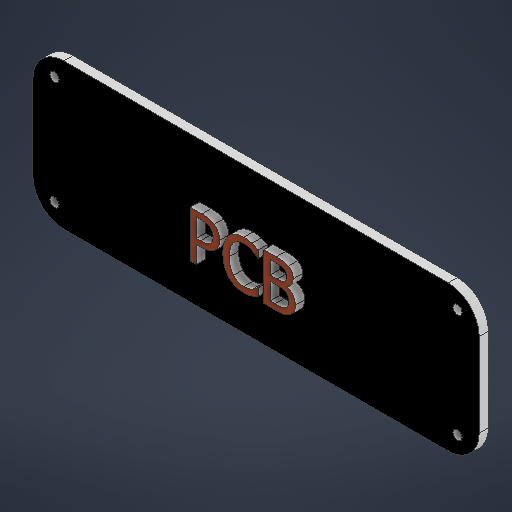
# Autodesk Inventor part: PCB
Saved by Autodesk Inventor 2025 (Build 290162000, 162)
## iProperties
Created: 2024-05-23
Part Number: PCB
Material: Generic
Document SubType Name: Modeling
Designer: techn
Density: 1 g/cm^3
Appearance: Default
Author: techn
Autodesk Inventor part; units mm, degrees
ref_plane "YZ Plane" through (0, 0, 0) normal (1, 0, 0) x (0, 1, 0)
ref_plane "XZ Plane" through (0, 0, 0) normal (0, 1, 0) x (-1, 0, 0)
ref_plane "XY Plane" through (0, 0, 0) normal (0, 0, 1) x (1, 0, 0)
sketch "Sketch1" plane through (0, 0, 0) normal (0, 0, 1) x (1, 0, 0)
  circle A0 centre (0, 0) radius 1.5
  circle A1 centre (0, 0) radius 3
  circle A2 centre (0, 35) radius 1.5
  circle A3 centre (0, 35) radius 3
  circle A4 centre (130, 35) radius 1.5
  circle A5 centre (130, 35) radius 3
  circle A6 centre (130, 0) radius 1.5
  circle A7 centre (130, 0) radius 3
  line L0 (3, 41) -> (127, 41)
  line L1 (137, 31) -> (137, 4)
  line L2 (127, -6) -> (3, -6)
  line L3 (-7, 4) -> (-7, 31)
  arc A8 (3, 41) -> (-7, 31) centre (3, 31) ccw
  arc A9 (-7, 4) -> (3, -6) centre (3, 4) ccw
  arc A10 (127, -6) -> (137, 4) centre (127, 4) ccw
  arc A11 (137, 31) -> (127, 41) centre (127, 31) ccw
  dimension "d0" = 3
  dimension "d1" = 1.5
  dimension "d2" = 3
  dimension "d3" = 1.5
  dimension "d4" = 3
  dimension "d5" = 1.5
  dimension "d6" = 3
  dimension "d7" = 1.5
  dimension "d8" = 130
  dimension "d9" = 35
  dimension "d10" = 7
  dimension "d11" = 6
  dimension "d12" = 6
  dimension "d13" = 7
  dimension "d14" = 10
  constraints: 12 centre point, 8 end point, 8 point on circle, 8 tangent, 3 equal radius, 2 horizontal alignment, 2 parallel, 2 vertical alignment, 1 coincident, 1 horizontal, 1 perpendicular
  measures "d0" diameter of A0
  measures "d1" radial gap between concentric circles of A0 A1
  measures "d2" diameter of A2
  measures "d3" radial gap between concentric circles of A2 A3
  measures "d4" diameter of A4
  measures "d5" radial gap between concentric circles of A4 A5
  measures "d6" diameter of A6
  measures "d7" radial gap between concentric circles of A6 A7
  measures "d8" distance of A6.centre A0.centre
  measures "d9" distance of A0.centre A2.centre
  measures "d10" distance from line of L3 A2.centre
  measures "d11" distance from line of L0 A2.centre
  measures "d12" distance from line of L2 A0.centre
  measures "d13" distance from line of L1 A6.centre
  measures "d14" radius of A8
extrude "Extrusion1" add sketch "Sketch1" along normal blind 3 contours A1 | A3 | A5 | A7 | L0 A11 L1 A10 L2 A9 L3 A8
sketch "Sketch2" plane through (0, 0, 3) normal (0, 0, 1) x (1, 0, 0)
  line L0 (45.2495, 23.7774) -> (59.8569, 23.7774) construction
  line L1 (59.8569, 23.7774) -> (59.8569, 17.4599) construction
  line L2 (59.8569, 17.4599) -> (45.2495, 17.4599) construction
  line L3 (45.2495, 17.4599) -> (45.2495, 23.7774) construction
  spline S0 degree 2 poles (56.2503, 18.9881) (56.2503, 18.0156) (55.5574, 16.2652) (54.9375, 15.6575) knots 0 0 0 1 2 2 2
  spline S1 degree 2 poles (54.9375, 15.6575) (54.1595, 14.8917) (52.0566, 14.1015) (50.4521, 14.1015) knots 0 0 0 1 2 2 2
  line L4 (50.4521, 14.1015) -> (48.7624, 14.1015)
  line L5 (48.7624, 14.1015) -> (48.7624, 8.51)
  line L6 (48.7624, 8.51) -> (46.7689, 8.51)
  line L7 (46.7689, 8.51) -> (46.7689, 23.51)
  line L8 (46.7689, 23.51) -> (50.5372, 23.51)
  spline S2 degree 2 poles (50.5372, 23.51) (51.8743, 23.51) (53.7462, 23.0724) (54.4634, 22.574) knots 0 0 0 1 2 2 2
  spline S3 degree 2 poles (54.4634, 22.574) (55.3022, 22.0027) (56.2503, 20.2401) (56.2503, 18.9881) knots 0 0 0 1 2 2 2
  spline S4 degree 2 poles (54.1717, 18.9273) (54.1717, 19.7053) (53.6368, 20.8479) (53.0898, 21.2126) knots 0 0 0 1 2 2 2
  spline S5 degree 2 poles (53.0898, 21.2126) (52.6158, 21.5286) (51.3516, 21.7839) (50.4156, 21.7839) knots 0 0 0 1 2 2 2
  line L9 (50.4156, 21.7839) -> (48.7624, 21.7839)
  line L10 (48.7624, 21.7839) -> (48.7624, 15.8033)
  line L11 (48.7624, 15.8033) -> (50.1239, 15.8033)
  spline S6 degree 2 poles (50.1239, 15.8033) (51.3394, 15.8033) (52.8346, 16.1923) (53.3208, 16.7028) knots 0 0 0 1 2 2 2
  spline S7 degree 2 poles (53.3208, 16.7028) (53.7705, 17.1526) (54.1717, 18.2101) (54.1717, 18.9273) knots 0 0 0 1 2 2 2
  spline S8 degree 2 poles (64.0056, 8.2425) (62.5469, 8.2425) (60.0793, 9.2271) (59.1798, 10.2117) knots 0 0 0 1 2 2 2
  spline S9 degree 2 poles (59.1798, 10.2117) (58.2803, 11.1842) (57.2957, 14.1015) (57.2957, 15.9978) knots 0 0 0 1 2 2 2
  spline S10 degree 2 poles (57.2957, 15.9978) (57.2957, 17.8819) (58.256, 20.6777) (59.1676, 21.7109) knots 0 0 0 1 2 2 2
  spline S11 degree 2 poles (59.1676, 21.7109) (60.0671, 22.7199) (62.5226, 23.7774) (64.042, 23.7774) knots 0 0 0 1 2 2 2
  spline S12 degree 2 poles (64.042, 23.7774) (64.7957, 23.7774) (66.1206, 23.5586) (66.6798, 23.3884) knots 0 0 0 1 2 2 2
  spline S13 degree 2 poles (66.6798, 23.3884) (67.166, 23.2304) (68.1749, 22.7806) (68.6733, 22.5132) knots 0 0 0 1 2 2 2
  line L12 (68.6733, 22.5132) -> (68.6733, 20.1064)
  line L13 (68.6733, 20.1064) -> (68.5153, 20.1064)
  spline S14 degree 2 poles (68.5153, 20.1064) (68.2479, 20.3495) (67.4213, 21.0302) (66.8257, 21.3584) knots 0 0 0 1 2 2 2
  spline S15 degree 2 poles (66.8257, 21.3584) (66.2543, 21.6745) (64.9051, 22.0756) (64.0299, 22.0756) knots 0 0 0 1 2 2 2
  spline S16 degree 2 poles (64.0299, 22.0756) (63.0696, 22.0756) (61.3556, 21.2855) (60.7114, 20.5318) knots 0 0 0 1 2 2 2
  spline S17 degree 2 poles (60.7114, 20.5318) (60.0793, 19.766) (59.3743, 17.4443) (59.3743, 15.9978) knots 0 0 0 1 2 2 2
  spline S18 degree 2 poles (59.3743, 15.9978) (59.3743, 14.4541) (60.1158, 12.2296) (60.76, 11.4638) knots 0 0 0 1 2 2 2
  spline S19 degree 2 poles (60.76, 11.4638) (61.3921, 10.7223) (63.0817, 9.9686) (64.0299, 9.9686) knots 0 0 0 1 2 2 2
  spline S20 degree 2 poles (64.0299, 9.9686) (64.8929, 9.9686) (66.3637, 10.3941) (66.9351, 10.7101) knots 0 0 0 1 2 2 2
  spline S21 degree 2 poles (66.9351, 10.7101) (67.4821, 11.0262) (68.2965, 11.6826) (68.5274, 11.9135) knots 0 0 0 1 2 2 2
  line L14 (68.5274, 11.9135) -> (68.6733, 11.9135)
  line L15 (68.6733, 11.9135) -> (68.6733, 9.531)
  spline S22 degree 2 poles (68.6733, 9.531) (68.1749, 9.3001) (67.2997, 8.8746) (66.6798, 8.6801) knots 0 0 0 1 2 2 2
  spline S23 degree 2 poles (66.6798, 8.6801) (66.0234, 8.4613) (64.9051, 8.2425) (64.0056, 8.2425) knots 0 0 0 1 2 2 2
  spline S24 degree 2 poles (80.7073, 13.1169) (80.7073, 11.9986) (79.8564, 10.2847) (79.1514, 9.7255) knots 0 0 0 1 2 2 2
  spline S25 degree 2 poles (79.1514, 9.7255) (78.3005, 9.0691) (76.3678, 8.51) (74.8362, 8.51) knots 0 0 0 1 2 2 2
  line L16 (74.8362, 8.51) -> (70.5331, 8.51)
  line L17 (70.5331, 8.51) -> (70.5331, 23.51)
  line L18 (70.5331, 23.51) -> (74.508, 23.51)
  spline S26 degree 2 poles (74.508, 23.51) (76.1125, 23.51) (77.7171, 23.3033) (78.4464, 22.9022) knots 0 0 0 1 2 2 2
  spline S27 degree 2 poles (78.4464, 22.9022) (79.2608, 22.4767) (80.0023, 21.0788) (80.0023, 20.1307) knots 0 0 0 1 2 2 2
  spline S28 degree 2 poles (80.0023, 20.1307) (80.0023, 19.0732) (78.884, 17.3957) (77.8994, 16.9216) knots 0 0 0 1 2 2 2
  line L19 (77.8994, 16.9216) -> (77.8994, 16.8487)
  spline S29 degree 2 poles (77.8994, 16.8487) (79.2365, 16.484) (80.7073, 14.5513) (80.7073, 13.1169) knots 0 0 0 1 2 2 2
  spline S30 degree 2 poles (78.6287, 13.0318) (78.6287, 13.8827) (78.1425, 14.9767) (77.4132, 15.3657) knots 0 0 0 1 2 2 2
  spline S31 degree 2 poles (77.4132, 15.3657) (76.9391, 15.6088) (75.8208, 15.7547) (74.7876, 15.7547) knots 0 0 0 1 2 2 2
  line L20 (74.7876, 15.7547) -> (72.5266, 15.7547)
  line L21 (72.5266, 15.7547) -> (72.5266, 10.2117)
  line L22 (72.5266, 10.2117) -> (74.1433, 10.2117)
  spline S32 degree 2 poles (74.1433, 10.2117) (75.4561, 10.2117) (76.9634, 10.4549) (77.5469, 10.8438) knots 0 0 0 1 2 2 2
  spline S33 degree 2 poles (77.5469, 10.8438) (78.106, 11.245) (78.6287, 12.2417) (78.6287, 13.0318) knots 0 0 0 1 2 2 2
  spline S34 degree 2 poles (77.9237, 19.8511) (77.9237, 20.386) (77.559, 21.1882) (77.1579, 21.4192) knots 0 0 0 1 2 2 2
  spline S35 degree 2 poles (77.1579, 21.4192) (76.6717, 21.6866) (75.4926, 21.8082) (74.4351, 21.8082) knots 0 0 0 1 2 2 2
  line L23 (74.4351, 21.8082) -> (72.5266, 21.8082)
  line L24 (72.5266, 21.8082) -> (72.5266, 17.42)
  line L25 (72.5266, 17.42) -> (74.7876, 17.42)
  spline S36 degree 2 poles (74.7876, 17.42) (75.7235, 17.42) (76.6109, 17.6145) (77.085, 17.9184) knots 0 0 0 1 2 2 2
  spline S37 degree 2 poles (77.085, 17.9184) (77.5469, 18.2101) (77.9237, 19.1461) (77.9237, 19.8511) knots 0 0 0 1 2 2 2
  point P0 (0, 0)
  dimension "d6" = 3
  constraints: 2 other
extrude "Extrusion2" add sketch "Sketch2" along normal blind 3
body "Solid1"
